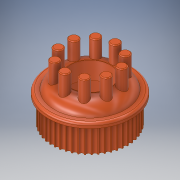
# Autodesk Inventor part: Orangatang Kegel Flat Face Adapter_2
Saved by Autodesk Inventor 2019.2 (Build 232265000, 265)
## iProperties
Created: 2018-11-27
Part Number: Orangatang Kegel Flat Face Adapter_2
Material: ABS Plastic
Document SubType Name: Modeling
Designer: Petar
Density: 1.06 g/cm^3
Appearance: Smooth - Light Orange
Author: Petar
Autodesk Inventor part; units mm, degrees
ref_plane "YZ Plane" through (0, 0, 0) normal (1, 0, 0) x (0, 1, 0)
ref_plane "XZ Plane" through (0, 0, 0) normal (0, 1, 0) x (-1, 0, 0)
ref_plane "XY Plane" through (0, 0, 0) normal (0, 0, 1) x (1, 0, 0)
sketch "Sketch1" plane through (0, 0, 0) normal (0, 1, 0) x (-1, 0, 0)
  circle A0 centre (0, 0) radius 22.4
  circle A1 centre (0, 0) radius 12.5
  dimension "d0" = 44.8
  dimension "d1" = 25
  constraints: 2 centre point, 2 coincident
  measures "d0" diameter of A0
  measures "d1" diameter of A1
extrude "Extrusion1" add sketch "Sketch1" along normal blind 7
fillet "Fillet1" radius 10 1 edges at (22.4, 7, 0)
sketch "Sketch2" plane through (0, 0, 0) normal (0, -1, 0) x (1, 0, 0)
  circle A0 centre (0, 0) radius 12.5 projected
  circle A1 centre (0, -15.85) radius 2.9
  dimension "d5" = 5.8
  dimension "d6" = 15.85
  constraints: 1 centre point
  measures "d5" diameter of A1
  measures "d6" distance of A0.centre A1.centre
extrude "Extrusion2" add sketch "Sketch2" against normal blind 18 contours A1
chamfer "Chamfer1" distance 0.5 angle 45 1 edges at (-2.9, 18, -15.85)
pattern_circular "Circular Pattern1" count 10 over 360 about axis through (0, 0, 0) along (0, 1, 0) of "Extrusion2", "Chamfer1"
ref_plane "Work Plane1" through (0, -20, 0) normal (0, -1, 0) x (1, 0, 0)
sketch "Sketch3" plane through (0, -20, 0) normal (0, -1, 0) x (1, 0, 0)
  circle A0 centre (0, -23.8732) radius 1.2
  line L0 (0, 0) -> (0, -23.8732) construction
  circle A1 centre (0, 0) radius 23.8732
  dimension "d16" = 2.4
  dimension "d17" = 23.8732
  constraints: 2 coincident, 2 end point, 1 centre point, 1 vertical alignment, 2 other
  measures "d16" diameter of A0
  measures "d17" distance of L0.start L0.end
sketch "Sketch4" plane through (0, 0, 0) normal (0, -1, 0) x (1, 0, 0)
  circle A0 centre (0, 0) radius 12.5 projected
  circle A1 centre (0, 0) radius 23.8732 projected
  circle A2 centre (0, 0) radius 26.2732
  dimension "d18" = 2.4
  constraints: 1 centre point, 1 coincident
  measures "d18" radial gap between concentric circles of A1 A2
extrude "Extrusion3" add sketch "Sketch4" along normal blind 4 contours A1 | A2
fillet "Fillet2" radius 1.5 1 edges at (-26.2732, 0, 0)
chamfer "Chamfer2" distance 2.4 distance2 1 1 edges at (-26.2732, -4, 0) measured on face at (-25.7732, -4, 0)
sketch "Sketch5" plane through (0, -4, 0) normal (0, -1, 0) x (1, 0, 0)
  circle A0 centre (0, 0) radius 12.5 projected
  circle A1 centre (0, -23.8732) radius 1.2 projected
  line L0 (0, 0) -> (0, -23.8732) construction
  circle A2 centre (0, 0) radius 23.8732 projected
  constraints: 1 vertical alignment
extrude "Extrusion4" add sketch "Sketch5" along normal blind 15 contours A2 A1 | A1 A2 picked at (-0.0474, -23.4738) picked at (19.7227, 2.9302)
extrude "Extrusion5" cut sketch "Sketch5" along normal through all contours A1 A2 | A2 A1 picked at (0.0436, -24.2686) picked at (-0.0474, -23.4738)
pattern_circular "Circular Pattern2" count 50 over 360 about axis through (0, 0, 0) along (0, 1, 0) of "Extrusion5"
chamfer "Chamfer3" distance 15 distance2 3 1 edges at (-12.5, -19, 0) measured on face at (-12.5, -18.5, 0)
sketch "Sketch6" plane through (0, -19, 0) normal (0, -1, 0) x (1, 0, 0)
  arc A0 (-21.0631, -11.2373) -> (-22.0846, -9.0664) centre (-21.6012, -10.1647) ccw projected
  circle A1 centre (0, 0) radius 15.5 projected
  circle A2 centre (0, 0) radius 17.5
  circle A3 centre (0, 0) radius 20.6732
  arc A4 (1.1996, -23.8431) -> (1.7982, -23.8054) centre (0, 0) ccw projected
  line L0 (1.25, -21.2619) -> (-1.25, -21.2619)
  line L1 (-1.25, -21.2619) -> (-1.25, -16.7619)
  line L2 (-1.25, -16.7619) -> (1.25, -16.7619)
  line L3 (1.25, -16.7619) -> (1.25, -21.2619)
  line L4 (0, 0) -> (0, -28) construction
  dimension "d35" = 2
  dimension "d36" = 2
  dimension "d42" = 2.5
  dimension "d43" = 4.5
  constraints: 10 end point, 2 centre point, 2 coincident, 2 parallel, 1 horizontal, 1 perpendicular, 1 vertical, 1 other
  measures "d36" radial gap between concentric circles of A2 A1
  measures "d42" distance of L1.end L2.end
  measures "d43" distance of L0.end L1.end
extrude "Extrusion6" cut sketch "Sketch6" against normal blind 15 contours A2 L1 A3 L3 | A2 L3 A3 L1
chamfer "Chamfer4" distance 15 distance2 2 1 edges at (-20.6732, -4, 0) measured on face at (-20.6732, -4.5, 0)
extrude "Extrusion7" add sketch "Sketch6" against normal blind 20 contours L1 L2 L3 A2 | A2 L3 A3 L1 | A3 L3 L0 L1 picked at (-0.139, -17.0063) picked at (0.9723, -18.5286)
pattern_circular "Circular Pattern3" count 20 over 360 about axis through (0, -11.5, 0) along (0, -1, 0) of "Extrusion7"
body "Solid1"
